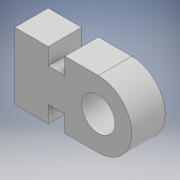
# Autodesk Inventor part: 32
Saved by Autodesk Inventor 2017 (Build 210142000, 142)
## iProperties
Part Number: 32
Material: 一般
Document SubType Name: Modeling
Designer: Brian
Density: 1 g/cm^3
Appearance: 預設
Mass: 42.2832 g
Surface Area: 103.416 cm^2
Volume: 42.2832 cm^3
Author: Brian
Autodesk Inventor part; units mm, degrees
ref_plane "YZ Plane" through (0, 0, 0) normal (1, 0, 0) x (0, 1, 0)
ref_plane "XZ Plane" through (0, 0, 0) normal (0, 1, 0) x (-1, 0, 0)
ref_plane "XY Plane" through (0, 0, 0) normal (0, 0, 1) x (1, 0, 0)
sketch "草圖1" plane through (0, 0, 0) normal (0, 1, 0) x (-1, 0, 0)
  line L0 (0, 0) -> (-70, 0)
  line L1 (-70, 0) -> (-70, -40)
  line L2 (-70, -40) -> (0, -40)
  line L3 (0, -40) -> (0, 0)
  dimension "d0" = 40
  dimension "d1" = 70
  constraints: 8 end point, 2 parallel, 1 horizontal, 1 perpendicular
  measures "d0" distance of L2.end L0.start
  measures "d1" distance of L1.end L2.end
extrude "擠出1" add sketch "草圖1" along normal blind 20
sketch "草圖2" plane through (0, 20, 0) normal (0, 1, 0) x (1, 0, 0)
  line L0 (0, 0) -> (70, 0) projected
  line L1 (20, 0) -> (30, 0)
  line L2 (30, 0) -> (30, 10)
  line L3 (30, 10) -> (20, 10)
  line L4 (20, 10) -> (20, 0)
  line L5 (70, 40) -> (0, 40) projected
  line L6 (20, 40) -> (30, 40)
  line L7 (30, 40) -> (30, 30)
  line L8 (30, 30) -> (20, 30)
  line L9 (20, 30) -> (20, 40)
  line L10 (0, 40) -> (0, 0) projected
  dimension "d4" = 10
  dimension "d5" = 10
  dimension "d6" = 10
  dimension "d7" = 20
  constraints: 16 end point, 4 parallel, 4 point on line, 2 horizontal, 2 perpendicular
  measures "d4" distance of L3.end L1.start
  measures "d5" distance of L8.end L6.start
  measures "d6" distance of L7.end L8.end
  measures "d7" distance between parallel lines of L10 L9
extrude "擠出2" cut sketch "草圖2" against normal blind 20
fillet "圓角1" radius 20 2 edges at (70, 10, 0) (70, 10, -40)
hole "孔1" at (50, 20, -20) direction (0, -1, 0) diameter 20 depth 20 tip angle 118
